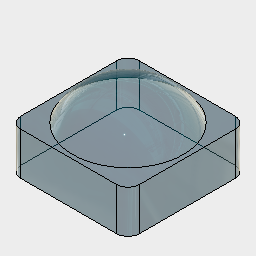
Mykroscope Cardboard (Autodesk Fusion 360 archive; units mm, degrees)
design "Magnifying Lens"
Autodesk Fusion 360 part; units mm, degrees
sketch "Sketch1" plane through (0, 0, 0) normal (0, 0, 1) x (1, 0, 0)
  line L0 (-5.15, 5.15) -> (5.15, 5.15)
  line L1 (5.15, 5.15) -> (5.15, -5.15)
  line L2 (5.15, -5.15) -> (-5.15, -5.15)
  line L3 (-5.15, -5.15) -> (-5.15, 5.15)
  dimension "d1" = 10.3
  dimension "d2" = 10.3
  dimension "d3" = 5.15
  dimension "d4" = 5.15
  measures "d1" distance of L0.start L0.end
  measures "d2" distance of L0.start L2.end
  measures "d3" distance of origin L3
  measures "d4" distance of origin L0
extrude "Extrude1" add sketch "Sketch1" along normal blind 3.7
sketch "Sketch2" plane through (0, 0, 0) normal (0, 1, 0) x (1, 0, 0)
  line L0 (-5.15, -3.7) -> (5.15, -3.7)
  line L1 (0, -3.7) -> (0, -6.6)
  line L2 (5.15, 0) -> (-5.15, 0)
  line L3 (0, -3.7) -> (4.8, -3.7)
  arc A0 (0, -6.6) -> (4.8, -3.7) centre (-0.149, -0.931) ccw
  dimension "d7" = 6.6
  dimension "d8" = 4.8
  measures "d7" distance of L1.end L2
  measures "d8" distance of L1.start L3.end
revolve "Revolve1" add sketch "Sketch2" angle 360 about axis through (0, 0, 3.7) along (0, 0, 1)
fillet "Fillet1" radius 1 4 edges at (5.15, -5.15, 1.85) (5.15, 5.15, 1.85) (-5.15, 5.15, 1.85) (-5.15, -5.15, 1.85)
equation "d3 = d1 / 2"
equation "d4 = d2 / 2"
equation "d8 = ( 9.6 / 2 ) * 1 mm"
